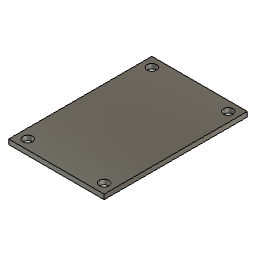
top plate v1 (Autodesk Fusion 360 design; units mm, degrees)
Autodesk Fusion 360 part; units mm, degrees
sketch "Sketch1" plane through (0, 0, 0) normal (0, 0, 1) x (1, 0, 0)
  line L0 (0, 0) -> (100, 0)
  line L1 (100, 0) -> (100, -150)
  line L2 (0, 0) -> (0, -150)
  line L3 (0, -150) -> (100, -150)
  dimension "d1" = 100
  dimension "d2" = 150
  constraint coincident L0.start L2.start
  constraint horizontal L0
  constraint perpendicular L0 L1
  constraint perpendicular L0 L2
  constraint perpendicular L1 L3
  measures "d1" distance of L0.start L0.end
  measures "d2" distance of L0.end L1.end
extrude "Extrude1" add sketch "Sketch1" along normal blind 5
hole "Hole1" at (10, -10, 5) direction (0, 0, -1) diameter 10 depth 5 tip angle 180
hole "Hole2" at (90, -10, 5) direction (0, 0, -1) diameter 10 depth 5 tip angle 180
hole "Hole3" at (10, -140, 5) direction (0, 0, -1) diameter 10 depth 5 tip angle 180
hole "Hole4" at (90, -140, 5) direction (0, 0, -1) diameter 10 depth 5 tip angle 180
